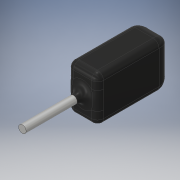
# Autodesk Inventor part: Netzwerk
Saved by Autodesk Inventor 2017 SP1 (Build 210196100, 196)
## iProperties
Part Number: Netzwerk
Material: Generisch
Document SubType Name: Modeling
Designer: Alex
Density: 1 g/cm^3
Appearance: Vorgabe
Author: Alex
Autodesk Inventor part; units mm, degrees
ref_plane "YZ Plane" through (0, 0, 0) normal (1, 0, 0) x (0, 1, 0)
ref_plane "XZ Plane" through (0, 0, 0) normal (0, 1, 0) x (-1, 0, 0)
ref_plane "XY Plane" through (0, 0, 0) normal (0, 0, 1) x (1, 0, 0)
sketch "Skizze2" plane through (0, 0, 0) normal (0, 1, 0) x (-1, 0, 0)
  line L0 (2, 3) -> (0, 3)
  line L1 (0, 3) -> (0, 0)
  line L2 (0, 0) -> (2, 0)
  line L3 (2, 0) -> (2, 3)
  dimension "d0" = 2
  dimension "breite" = 3
  constraints: 8 end point, 2 parallel, 1 coincident, 1 horizontal, 1 perpendicular
  measures "d0" distance of L2.end L1.end
  measures "breite" distance of L1.end L0.end
extrude "Extrusion1" add sketch "Skizze2" along normal blind 5
sketch "Skizze3" plane through (0, 0, 0) normal (0, -1, 0) x (1, 0, 0)
  circle A0 centre (-1, 1.5) radius 0.25
  line L0 (0, 0) -> (-2, 0) projected
  line L1 (0, 3) -> (0, 0) projected
  dimension "d4" = 0.5
  dimension "BeinPos" = 1.5
  dimension "d6" = 1
  constraints: 1 centre point
  measures "d4" diameter of A0
  measures "BeinPos" distance from line of L0 A0.centre
  measures "d6" distance from line of L1 A0.centre
extrude "Extrusion2" add sketch "Skizze3" along normal blind 4
fillet "Rundung2" radius 0.6 1 edges at (-1.25, 0, 1.5)
fillet "Rundung3" radius 0.4 4 edges at (0, 2.5, 0) (0, 2.5, 3) (-2, 2.5, 3) (-2, 2.5, 0)
fillet "Rundung4" radius 0.9 8 edges at (0, 5, 1.5) (-0.1172, 5, 0.1172) (-1, 5, 0) (-1.8828, 5, 0.1172) (-2, 5, 1.5) (-1.8828, 5, 2.8828) (-1, 5, 3) (-0.1172, 5, 2.8828)
fillet "Rundung5" radius 0.4 8 edges at (0, 0, 1.5) (-0.1172, 0, 0.1172) (-1, 0, 0) (-1.8828, 0, 0.1172) (-2, 0, 1.5) (-1.8828, 0, 2.8828) (-1, 0, 3) (-0.1172, 0, 2.8828)
equation "\"BeinPos\" = 0.5 * breite"
